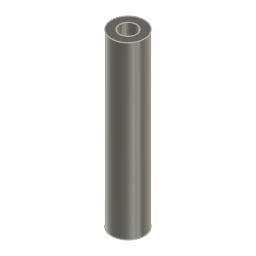
link piece (Autodesk Fusion 360 design; units mm, degrees)
Autodesk Fusion 360 part; units mm, degrees
sketch "Sketch1" plane through (0, 0, 0) normal (0, 0, 1) x (1, 0, 0)
  line L0 (-3.8105, 0) -> (-1.9053, -3.3)
  line L1 (-1.9053, -3.3) -> (1.9053, -3.3)
  line L2 (1.9053, -3.3) -> (3.8105, 0)
  line L3 (3.8105, 0) -> (1.9053, 3.3)
  line L4 (1.9053, 3.3) -> (-1.9053, 3.3)
  line L5 (-1.9053, 3.3) -> (-3.8105, 0)
  circle A0 centre (0, 0) radius 4.75
  dimension "d1" = 3.3
  dimension "d12" = 9.5
  constraint coincident A0.centre origin
  constraint horizontal L1
  measures "d1" distance of A0.centre L5
  measures "d12" diameter of A0
extrude "Extrude1" add sketch "Sketch1" along normal blind 13
sketch "Sketch4" plane through (0, 0, 13) normal (0, 0, 1) x (-1, 0, 0)
  line L0 (3.8105, 0) -> (1.9053, -3.3)
  line L1 (1.9053, -3.3) -> (-1.9053, -3.3)
  line L2 (-1.9053, -3.3) -> (-3.8105, 0)
  line L3 (-3.8105, 0) -> (-1.9053, 3.3)
  line L4 (-1.9053, 3.3) -> (1.9053, 3.3)
  line L5 (1.9053, 3.3) -> (3.8105, 0)
  circle A0 centre (0, 0) radius 4.75
extrude "Extrude2" add sketch "Sketch4" along normal blind 2 contours L0 L1 L2 L3 L4 L5 | A0
sketch "Sketch3" plane through (0, 0, 15) normal (0, 0, 1) x (-1, 0, 0)
  circle A0 centre (0, 0) radius 2.45
  circle A1 centre (0, 0) radius 4.75
  dimension "d7" = 4.9
  constraint coincident A0.centre A1.centre
  measures "d7" diameter of A0
extrude "Extrude5" add sketch "Sketch3" along normal blind 38.2
move_face "OffsetFaces1" offset -4 1 faces at (-3.2135, 1.9919, 0)
equation "d13 = 38.3 mm + 0.8 mm - 0.9 mm"
named bodies: "link left"
